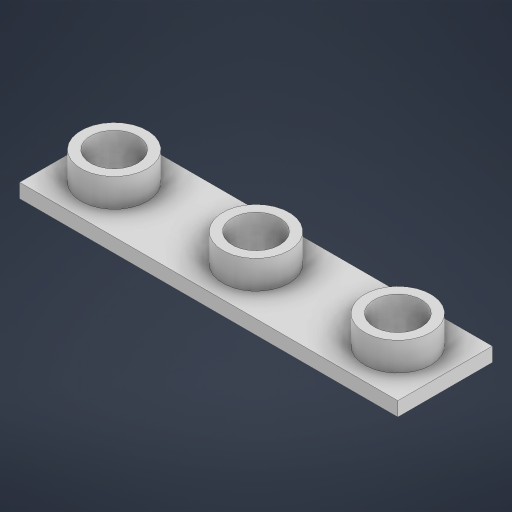
# Autodesk Inventor part: GANJEL LED
Saved by Autodesk Inventor 2024 (Build 280153000, 153)
## iProperties
Created: 2025-06-24
Part Number: GANJEL LED
Material: Generic
Document SubType Name: Modeling
Designer: ASUS
Density: 1 g/cm^3
Appearance: Default
Author: ASUS
Autodesk Inventor part; units mm, degrees
ref_plane "YZ Plane" through (0, 0, 0) normal (1, 0, 0) x (0, 1, 0)
ref_plane "XZ Plane" through (0, 0, 0) normal (0, 1, 0) x (-1, 0, 0)
ref_plane "XY Plane" through (0, 0, 0) normal (0, 0, 1) x (1, 0, 0)
sketch "Sketch1" plane through (0, 0, 0) normal (0, 1, 0) x (-1, 0, 0)
  line L0 (20, -5) -> (-20, -5)
  line L1 (-20, -5) -> (-20, 5)
  line L2 (-20, 5) -> (20, 5)
  line L3 (20, 5) -> (20, -5)
  circle A0 centre (0, 0) radius 2.5
  line L4 (0, 0) -> (15, 0)
  circle A1 centre (15, 0) radius 2.5
  line L5 (0, 0) -> (-15, 0)
  circle A2 centre (-15, 0) radius 2.5
  dimension "d0" = 40
  dimension "d1" = 10
  dimension "d13" = 5
  dimension "d14" = 15
  dimension "d15" = 5
  dimension "d16" = 15
  dimension "d17" = 5
  constraints: 12 end point, 3 centre point, 3 horizontal, 2 coincident, 2 parallel, 1 perpendicular
  measures "d0" distance of L1.end L2.end
  measures "d1" distance of L0.end L1.end
  measures "d13" diameter of A0
  measures "d14" distance of L4.start L4.end
  measures "d15" diameter of A1
  measures "d16" distance of L4.start L5.end
  measures "d17" diameter of A2
extrude "Extrusion1" add sketch "Sketch1" along normal blind 1.5
sketch "Sketch4" plane through (0, 1.5, 0) normal (0, 1, 0) x (1, 0, 0)
  circle A0 centre (0, 0) radius 3.5
  circle A1 centre (-15, 0) radius 3.5
  circle A2 centre (15, 0) radius 3.5
  circle A3 centre (-15, 0) radius 2.5
  circle A4 centre (0, 0) radius 2.5
  circle A5 centre (15, 0) radius 2.5
  dimension "d18" = 7
  dimension "d21" = 7
  dimension "d22" = 7
  dimension "d23" = 1
  dimension "d24" = 1
  dimension "d25" = 1
  constraints: 6 centre point, 1 coincident
  measures "d18" diameter of A0
  measures "d21" diameter of A1
  measures "d22" diameter of A2
  measures "d23" radial gap between concentric circles of A1 A3
  measures "d24" radial gap between concentric circles of A0 A4
  measures "d25" radial gap between concentric circles of A2 A5
extrude "Extrusion3" add sketch "Sketch4" along normal blind 3
body "Solid1"
